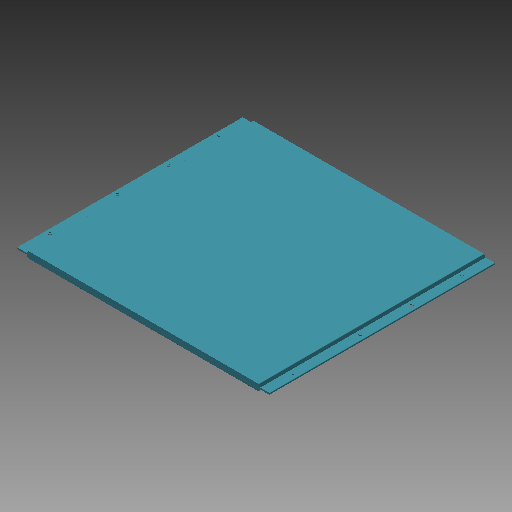
# Autodesk Inventor part: Tapicerka_oparcia
Saved by Autodesk Inventor 2017 (Build 210142000, 142)
## iProperties
Created: 2015-12-07
Part Number: Tapicerka_oparcia
Material: Nylon 6/6
Document SubType Name: Modeling
Designer: graaapsik
Density: 1.13 g/cm^3
Appearance: Niebieska z odcieniem szarości
Mass: 232.575 g
Surface Area: 7478.71 cm^2
Volume: 205.819 cm^3
Author: graaapsik
Autodesk Inventor part; units mm, degrees
ref_plane "YZ Plane" through (0, 0, 0) normal (1, 0, 0) x (0, 1, 0)
ref_plane "XZ Plane" through (0, 0, 0) normal (0, 1, 0) x (-1, 0, 0)
ref_plane "XY Plane" through (0, 0, 0) normal (0, 0, 1) x (1, 0, 0)
sketch "Szkic1" plane through (0, 0, 0) normal (0, 0, 1) x (1, 0, 0)
  line L0 (0, 0) -> (17.1, 0)
  line L1 (19.5, -4.25) -> (429, -4.25)
  line L2 (431.4, 0) -> (448.5, 0)
  line L3 (448.5, 0) -> (448.5, 3)
  line L4 (448.5, 3) -> (431.4, 3)
  line L5 (429, 7.25) -> (19.5, 7.25)
  line L6 (17.1, 3) -> (0, 3)
  line L7 (0, 3) -> (0, 0)
  line L8 (17.1, 0) -> (17.5, 1)
  line L9 (17.5, 1) -> (19.5, -4.25)
  line L10 (17.1, 3) -> (17.5, 2)
  line L11 (17.5, 2) -> (19.5, 7.25)
  line L12 (429, -4.25) -> (431, 1)
  line L13 (431, 1) -> (431.4, 0)
  line L14 (429, 7.25) -> (431, 2)
  line L15 (431, 2) -> (431.4, 3)
  line L16 (0, 1.5) -> (2.0282, 1.5) construction
  dimension "d1" = 17.5
  dimension "d2" = 1
  dimension "d3" = 1
  dimension "d4" = 3
  dimension "d5" = 17.5
  dimension "d6" = 448.5
  dimension "d7" = 11.5
  dimension "d10" = 2
  dimension "d11" = 0.4
  dimension "d12" = 2
  dimension "d38" = 0.4
  constraints: 34 end point, 5 horizontal, 4 equal length, 2 collinear, 2 vertical alignment, 1 midpoint, 1 perpendicular, 3 other
  measures "d1" horizontal distance of L8.end L0.start
  measures "d2" distance of L8.end L10.end
  measures "d3" distance of L12.end L14.end
  measures "d4" distance of L6.end L0.start
  measures "d5" distance from line of L3 L12.end
  measures "d6" distance between parallel lines of L3 L7
  measures "d7" distance between parallel lines of L1 L5
  measures "d10" horizontal distance of L5.end L10.end
  measures "d11" horizontal distance of L4.end L14.end
  measures "d12" horizontal distance of L5.start L14.end
  measures "d38" horizontal distance of L6.start L10.end
extrude "Wyciągnięcie proste1" add sketch "Szkic1" along normal mid plane 400
shell "Skorupa1" thickness 0.55 removed faces 2 at (292.5, -0.4167, 200) at (292.5, -0.4167, -200)
fillet "Zaokrąglenie1" radius 1 12 edges at (0, 3, 0) (0, 0, 0) (17.1, 3, 0) (17.1, 0, 0) (448.5, 0, 0) (448.5, 3, 0) (431.4, 0, 0) (431.4, 3, 0) (429, -4.25, 0) (429, 7.25, 0) (19.5, -4.25, 0) (19.5, 7.25, 0)
fillet "Zaokrąglenie3" radius 0.1 4 edges at (17.5, 2, 0) (17.5, 1, 0) (431, 2, 0) (431, 1, 0)
sketch "Szkic3" plane through (0, 0, 200) normal (0, 0, 1) x (1, 0, 0)
  line L0 (431.3924, 1.5) -> (431.7724, 2.45) projected
  line L1 (431.7724, 2.45) -> (447.95, 2.45) projected
  line L2 (447.95, 2.45) -> (447.95, 0.55) projected
  line L3 (447.95, 0.55) -> (431.7724, 0.55) projected
  line L4 (431.7724, 0.55) -> (431.3924, 1.5) projected
  line L5 (17.8981, 1.5) -> (19.879, 6.7) projected
  line L6 (19.879, 6.7) -> (428.621, 6.7) projected
  line L7 (428.621, 6.7) -> (430.6019, 1.5) projected
  line L8 (430.6019, 1.5) -> (428.621, -3.7) projected
  line L9 (428.621, -3.7) -> (19.879, -3.7) projected
  line L10 (19.879, -3.7) -> (17.8981, 1.5) projected
  line L11 (0.55, 0.55) -> (0.55, 2.45) projected
  line L12 (0.55, 2.45) -> (16.7276, 2.45) projected
  line L13 (16.7276, 2.45) -> (17.1076, 1.5) projected
  line L14 (17.1076, 1.5) -> (16.7276, 0.55) projected
  line L15 (16.7276, 0.55) -> (0.55, 0.55) projected
  point P0 (0, 0)
extrude "Wyciągnięcie proste3" add sketch "Szkic3" against normal blind 0.55
sketch "Szkic4" plane through (0, 0, -200) normal (0, 0, -1) x (-1, 0, 0)
  line L0 (-431.7724, 2.45) -> (-431.3924, 1.5) projected
  line L1 (-431.3924, 1.5) -> (-431.7724, 0.55) projected
  line L2 (-431.7724, 0.55) -> (-447.95, 0.55) projected
  line L3 (-447.95, 0.55) -> (-447.95, 2.45) projected
  line L4 (-447.95, 2.45) -> (-431.7724, 2.45) projected
  line L5 (-19.879, 6.7) -> (-17.8981, 1.5) projected
  line L6 (-17.8981, 1.5) -> (-19.879, -3.7) projected
  line L7 (-19.879, -3.7) -> (-428.621, -3.7) projected
  line L8 (-428.621, -3.7) -> (-430.6019, 1.5) projected
  line L9 (-430.6019, 1.5) -> (-428.621, 6.7) projected
  line L10 (-428.621, 6.7) -> (-19.879, 6.7) projected
  line L11 (-0.55, 2.45) -> (-0.55, 0.55) projected
  line L12 (-0.55, 0.55) -> (-16.7276, 0.55) projected
  line L13 (-16.7276, 0.55) -> (-17.1076, 1.5) projected
  line L14 (-17.1076, 1.5) -> (-16.7276, 2.45) projected
  line L15 (-16.7276, 2.45) -> (-0.55, 2.45) projected
  point P0 (0, 0)
extrude "Wyciągnięcie proste4" add sketch "Szkic4" against normal blind 0.55
fillet "Zaokrąglenie4" radius 0.1 56 edges at (19.6217, -4.0734, -200) (18.4229, -1.4227, -200) (17.4986, 0.8251, -200) (17.3782, 0.6954, -200) (16.9836, 0.1719, -200) (8.7115, 0, -200) (0.2929, 0.2929, -200) (8.7115, 3, -200) (16.9836, 2.8281, -200) (17.3782, 2.3046, -200) (17.4986, 2.1749, -200) (18.4229, 4.4227, -200) (19.6217, 7.0734, -200) (224.25, 7.25, -200) (428.8783, 7.0734, -200) (430.0771, 4.4227, -200) (431.0014, 2.1749, -200) (431.1218, 2.3046, -200) (431.5164, 2.8281, -200) (439.7885, 3, -200) (448.2071, 0.2929, -200) (439.7885, 0, -200) (431.5164, 0.1719, -200) (431.1218, 0.6954, -200) (431.0014, 0.8251, -200) (430.0771, -1.4227, -200) (428.8783, -4.0734, -200) (224.25, -4.25, -200) (19.6217, 7.0734, 200) (18.4229, 4.4227, 200) (17.4986, 2.1749, 200) (17.3782, 2.3046, 200) (16.9836, 2.8281, 200) (8.7115, 3, 200) (0.2929, 0.2929, 200) (8.7115, 0, 200) (16.9836, 0.1719, 200) (17.3782, 0.6954, 200) (17.4986, 0.8251, 200) (18.4229, -1.4227, 200) (19.6217, -4.0734, 200) (224.25, -4.25, 200) (428.8783, -4.0734, 200) (430.0771, -1.4227, 200) (431.0014, 0.8251, 200) (431.1218, 0.6954, 200) (431.5164, 0.1719, 200) (439.7885, 0, 200) (448.2071, 0.2929, 200) (439.7885, 3, 200) (431.5164, 2.8281, 200) (431.1218, 2.3046, 200) (431.0014, 2.1749, 200) (430.0771, 4.4227, 200) (428.8783, 7.0734, 200) (224.25, 7.25, 200)
sketch "Szkic5" plane through (0, 0, 0) normal (0, 1, 0) x (-1, 0, 0)
  line L0 (-448.5, -191.9) -> (-448.5, 191.9) construction
  line L1 (-448.5, 0) -> (0, 0) construction
  line L2 (-224.25, 0) -> (-224.25, 0) construction
  line L3 (-16.6615, -200) -> (-0.7615, -200) construction
  line L4 (-8.7115, -200) -> (-8.7115, 200) construction
  line L5 (-1, 200) -> (-16.423, 200) construction
  line L6 (-15.923, -200) -> (-1.5, -200)
  line L7 (-1, 200) -> (-16.423, 200) projected
  line L8 (-16.423, -200) -> (-1, -200) construction
  point P0 (-8.7115, -150)
  point P1 (-8.7115, -60)
  point P2 (-8.7115, 30)
  point P3 (-8.7115, 150)
  point P4 (-16.6615, -200)
  point P5 (-16.6615, -200)
  point P6 (-439.7885, -150)
  point P7 (-439.7885, -60)
  point P8 (-439.7885, 30)
  point P9 (-439.7885, 150)
  dimension "d26" = 15.9
  dimension "d27" = 50
  dimension "d28" = 50
  dimension "d29" = 90
  dimension "d30" = 90
  constraints: 14 end point, 4 midpoint, 4 symmetric about line, 3 perpendicular, 3 vertical alignment, 2 collinear, 1 horizontal, 1 point on line, 4 other
  measures "d26" distance of L3.start L3.end
  measures "d27" distance from line of point (-8.711, 150) L5
  measures "d28" distance from line of point (-8.711, -150) L6
  measures "d29" distance of point (-8.711, -60) point (-8.711, -150)
  measures "d30" distance of point (-8.711, 30) point (-8.711, -60)
hole "Otwór2" at (8.7115, 0, -150) at (8.7115, 0, -60) at (8.7115, 0, 30) at (8.7115, 0, 150) at (439.7885, 0, -150) at (439.7885, 0, -60) at (439.7885, 0, 30) at (439.7885, 0, 150) direction (0, 1, 0) diameter 6 end through all
